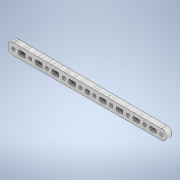
# Autodesk Inventor part: カウンター 中間部
Saved by Autodesk Inventor 2020.2 (Build 242310000, 310)
## iProperties
Created: 2020-05-03
Part Number: カウンター 中間部
Material: アルミニウム 7075
Document SubType Name: Modeling
Designer: mozar
Density: 2.81 g/cm^3
Appearance: サテン - ブラシ仕上げ 重厚
Mass: 15.7202 g
Surface Area: 50.7273 cm^2
Volume: 5.59439 cm^3
Author: mozar
Autodesk Inventor part; units mm, degrees
ref_plane "YZ Plane" through (0, 0, 0) normal (1, 0, 0) x (0, 1, 0)
ref_plane "XZ Plane" through (0, 0, 0) normal (0, 1, 0) x (-1, 0, 0)
ref_plane "XY Plane" through (0, 0, 0) normal (0, 0, 1) x (1, 0, 0)
sketch "スケッチ1" plane through (0, 0, 0) normal (0, 0, 1) x (1, 0, 0)
  line L0 (0, 0) -> (132.465, 0) construction
  line L1 (0, -5) -> (132.465, -5)
  line L2 (132.465, 5) -> (0, 5)
  arc A0 (0, 5) -> (0, -5) centre (0, 0) ccw
  arc A1 (132.465, -5) -> (132.465, 5) centre (132.465, 0) ccw
  circle A2 centre (132.465, 0) radius 4.5
  circle A3 centre (0, 0) radius 5
  line L3 (0.0189, 5) -> (132.482, 4.5)
  line L4 (132.482, -4.5) -> (0.0189, -5)
  point P0 (66.2325, 0)
  point P1 (15, 0)
  point P2 (30, 0)
  point P3 (72.465, 0)
  point P4 (87.465, 0)
  point P5 (102.465, 0)
  point P6 (117.465, 0)
  point P7 (45, 0)
  point P8 (60, 0)
  dimension "d0" = 132.465
  dimension "d1" = 10
  dimension "d2" = 9
  dimension "d3" = 10
  dimension "d4" = 15
  dimension "d5" = 15
  dimension "d6" = 15
  dimension "d7" = 15
  dimension "d8" = 15
  dimension "d9" = 15
  dimension "d10" = 15
  dimension "d11" = 15
  constraints: 8 end point, 8 point on circle, 8 tangent, 4 centre point, 2 coincident, 1 parallel, 14 other
  measures "d0" distance of A0.centre A1.centre
  measures "d1" diameter of A1
  measures "d2" diameter of A2
  measures "d3" diameter of A3
  measures "d4" distance of point (117.465, 0) A1.centre
  measures "d5" distance of point (102.465, 0) point (117.465, 0)
  measures "d6" distance of point (87.465, 0) point (102.465, 0)
  measures "d7" distance of point (87.465, 0) point (72.465, 0)
  measures "d8" distance of A0.centre point (15, 0)
  measures "d9" distance of point (15, 0) point (30, 0)
  measures "d10" distance of point (30, 0) point (45, 0)
  measures "d11" distance of point (45, 0) point (60, 0)
extrude "押し出し1" add sketch "スケッチ1" against normal blind 5 contours A0 L2 A3 L1 | A3 L3 A2 L4 | A2
hole "穴1" at (15, 0, 0) at (30, 0, 0) at (72.465, 0, 0) at (87.465, 0, 0) at (102.465, 0, 0) at (117.465, 0, 0) at (45, 0, 0) at (60, 0, 0) at (132.465, 0, 0) at (0, 0, 0) direction (0, 0, -1) diameter 3 depth 12 tip angle 118
sketch "スケッチ2" plane through (0, 0, 0) normal (0, 0, 1) x (1, 0, 0)
  circle A0 centre (132.465, 0) radius 1.5 projected
  circle A1 centre (45, 0) radius 1.5 projected
  circle A2 centre (102.465, 0) radius 1.5 projected
  circle A3 centre (72.465, 0) radius 1.5 projected
  circle A4 centre (15, 0) radius 1.5 projected
  circle A5 centre (30, 0) radius 1.5 projected
  circle A6 centre (87.465, 0) radius 1.5 projected
  circle A7 centre (117.465, 0) radius 1.5 projected
  circle A8 centre (60, 0) radius 1.5 projected
  circle A9 centre (0, 0) radius 1.5 projected
  line L0 (132.482, -4.5) -> (0.0189, -5) projected
  arc A10 (0.0189, 5) -> (0.0189, -5) centre (0, 0) ccw projected
  line L1 (0.0189, 5) -> (132.482, 4.5) projected
  arc A11 (132.482, -4.5) -> (132.482, 4.5) centre (132.465, 0) ccw projected
sketch "スケッチ3" plane through (0, 0, 0) normal (0, 0, 1) x (1, 0, 0)
  circle A0 centre (132.465, 0) radius 1.5 projected
  circle A1 centre (45, 0) radius 1.5 projected
  circle A2 centre (102.465, 0) radius 1.5 projected
  circle A3 centre (72.465, 0) radius 1.5 projected
  circle A4 centre (15, 0) radius 1.5 projected
  circle A5 centre (30, 0) radius 1.5 projected
  circle A6 centre (87.465, 0) radius 1.5 projected
  circle A7 centre (117.465, 0) radius 1.5 projected
  circle A8 centre (60, 0) radius 1.5 projected
  circle A9 centre (0, 0) radius 1.5 projected
  line L0 (132.482, -4.5) -> (0.0189, -5) projected
  arc A10 (0.0189, 5) -> (0.0189, -5) centre (0, 0) ccw projected
  line L1 (0.0189, 5) -> (132.482, 4.5) projected
  arc A11 (132.482, -4.5) -> (132.482, 4.5) centre (132.465, 0) ccw projected
  line L2 (132.4707, 1.5) -> (0.0075, 2)
  arc A12 (0.0075, 2) -> (0.0075, -2) centre (0, 0) ccw
  line L3 (0.0075, -2) -> (132.4707, -1.5)
  arc A13 (132.4707, -1.5) -> (132.4707, 1.5) centre (132.465, 0) ccw
  circle A14 centre (0, 0) radius 4.5
  circle A15 centre (15, 0) radius 4.5
  circle A16 centre (30, 0) radius 4.5
  circle A17 centre (45, 0) radius 4.5
  circle A18 centre (60, 0) radius 4.5
  circle A19 centre (72.465, 0) radius 4.5
  circle A20 centre (87.465, 0) radius 4.5
  circle A21 centre (102.465, 0) radius 4.5
  circle A22 centre (117.465, 0) radius 4.5
  circle A23 centre (132.465, 0) radius 4.5
  point P0 (98.2702, -1.6291)
  point P1 (98.2702, 1.6291)
  point P2 (91.65, 1.6541)
  point P3 (91.65, -1.6541)
  point P4 (113.2487, -1.5725)
  point P5 (113.2487, 1.5725)
  point P6 (106.6719, 1.5974)
  point P7 (106.6719, -1.5974)
  point P8 (128.2281, -1.516)
  point P9 (128.2281, 1.516)
  point P10 (121.693, 1.5407)
  point P11 (121.693, -1.5407)
  point P12 (83.2926, -1.6856)
  point P13 (83.2926, 1.6856)
  point P14 (76.6271, 1.7108)
  point P15 (76.6271, -1.7108)
  point P16 (68.3159, -1.7421)
  point P17 (68.3159, 1.7421)
  point P18 (64.1424, 1.7579)
  point P19 (64.1424, -1.7579)
  point P20 (55.871, -1.7891)
  point P21 (55.871, 1.7891)
  point P22 (49.1179, 1.8146)
  point P23 (49.1179, -1.8146)
  point P24 (40.8959, -1.8456)
  point P25 (40.8959, 1.8456)
  point P26 (34.0924, 1.8713)
  point P27 (34.0924, -1.8713)
  point P28 (25.9218, -1.9022)
  point P29 (25.9218, 1.9022)
  point P30 (19.066, 1.928)
  point P31 (19.066, -1.928)
  point P32 (10.9486, -1.9587)
  point P33 (10.9486, 1.9587)
  point P34 (4.0386, 1.9848)
  point P35 (4.0386, -1.9848)
  dimension "d21" = 3
  dimension "d22" = 3
  dimension "d23" = 3
  dimension "d24" = 3
  dimension "d25" = 3
  dimension "d26" = 3
  dimension "d27" = 3
  dimension "d28" = 3
  dimension "d29" = 3
  dimension "d30" = 3
  dimension "d31" = 3
  constraints: 12 centre point, 4 end point, 4 point on circle, 3 other
  measures "d21" distance between parallel lines of L1 L2
  measures "d22" radial gap between concentric circles of A9 A14
  measures "d23" radial gap between concentric circles of A4 A15
  measures "d24" radial gap between concentric circles of A5 A16
  measures "d25" radial gap between concentric circles of A1 A17
  measures "d26" radial gap between concentric circles of A8 A18
  measures "d27" radial gap between concentric circles of A3 A19
  measures "d28" radial gap between concentric circles of A6 A20
  measures "d29" radial gap between concentric circles of A2 A21
  measures "d30" radial gap between concentric circles of A7 A22
  measures "d31" radial gap between concentric circles of A0 A23
extrude "押し出し2" cut sketch "スケッチ3" against normal blind 4 contours A23 L3 A22 L2 | A22 L3 A21 L2 | A21 L3 A20 L2 | A20 L3 A19 L2 | A19 L3 A18 L2 | A18 L3 A17 L2 | A17 L3 A16 L2 | A16 L3 A15 L2 | A15 L3 A14 L2
fillet "フィレット1" radius 1 36 edges at (4.0386, -1.9848, -2) (4.0386, 1.9848, -2) (10.9486, 1.9587, -2) (10.9486, -1.9587, -2) (19.066, -1.928, -2) (19.066, 1.928, -2) (25.9218, 1.9022, -2) (25.9218, -1.9022, -2) (40.8959, 1.8456, -2) (40.8959, -1.8456, -2) (34.0924, 1.8713, -2) (34.0924, -1.8713, -2) (55.871, 1.7891, -2) (55.871, -1.7891, -2) (49.1179, 1.8146, -2) (49.1179, -1.8146, -2) (68.3159, 1.7421, -2) (68.3159, -1.7421, -2) (64.1424, 1.7579, -2) (64.1424, -1.7579, -2) (83.2926, 1.6856, -2) (83.2926, -1.6856, -2) (76.6271, 1.7108, -2) (76.6271, -1.7108, -2) (98.2702, 1.6291, -2) (98.2702, -1.6291, -2) (91.65, 1.6541, -2) (91.65, -1.6541, -2) (113.2487, 1.5725, -2) (113.2487, -1.5725, -2) (106.6719, 1.5974, -2) (106.6719, -1.5974, -2) (128.2281, 1.516, -2) (128.2281, -1.516, -2) (121.693, 1.5407, -2) (121.693, -1.5407, -2)
equation "\"d5\" = d4"
equation "\"d6\" = d4"
equation "\"d7\" = d4"
equation "\"d8\" = d4"
equation "\"d9\" = d4"
equation "\"d10\" = d4"
equation "\"d11\" = d4"
